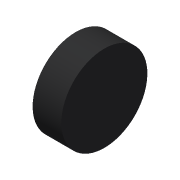
# Autodesk Inventor part: Wheel
Saved by Autodesk Inventor 2019 (Build 230136000, 136)
## iProperties
Created: 2019-04-28
Part Number: Wheel
Material: 고무
Document SubType Name: Modeling
Designer: hinmo
Mass: 1093.71 g
Surface Area: 712.749 cm^2
Volume: 1176.04 cm^3
Density: 0.93 g/cm^3
Appearance: 고무 - 검은색
Author: hinmo
Autodesk Inventor part; units mm, degrees
ref_plane "YZ Plane" through (0, 0, 0) normal (1, 0, 0) x (0, 1, 0)
ref_plane "XZ Plane" through (0, 0, 0) normal (0, 1, 0) x (-1, 0, 0)
ref_plane "XY Plane" through (0, 0, 0) normal (0, 0, 1) x (1, 0, 0)
sketch "스케치2" plane through (0, 0, 0) normal (1, 0, 0) x (0, 1, 0)
  circle A0 centre (0, 0) radius 82.5
  dimension "d0" = 165
  constraints: 1 centre point, 1 coincident
  measures "d0" diameter of A0
extrude "돌출1" add sketch "스케치2" along normal blind 55
